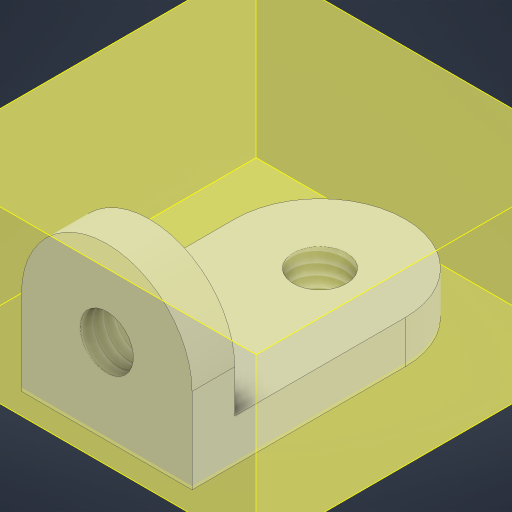
# Autodesk Inventor part: Rotational Linkage
Saved by Autodesk Inventor 2023 (Build 270158000, 158)
## iProperties
Created: 2022-05-02
Part Number: Rotational Linkage
Material: Generic
Document SubType Name: Modeling
Designer: FizzyApple12
Density: 1 g/cm^3
Appearance: Default
Author: FizzyApple12
Autodesk Inventor part; units mm, degrees
ref_plane "YZ Plane" through (0, 0, 0) normal (1, 0, 0) x (0, 1, 0)
ref_plane "XZ Plane" through (0, 0, 0) normal (0, 1, 0) x (-1, 0, 0)
ref_plane "XY Plane" through (0, 0, 0) normal (0, 0, 1) x (1, 0, 0)
sketch "Sketch1" plane through (0, 0, 0) normal (0, 1, 0) x (-1, 0, 0)
  circle A0 centre (0, 0) radius 6.35
  line L0 (6.35, 0) -> (6.35, 12.7)
  line L1 (6.35, 12.7) -> (-6.35, 12.7)
  line L2 (-6.35, 12.7) -> (-6.35, 0)
  dimension "d0" = 12.7
  dimension "d1" = 12.7
  constraints: 6 end point, 2 coincident, 2 point on circle, 2 tangent, 1 centre point, 1 parallel, 1 perpendicular, 1 vertical
  measures "d0" diameter of A0
  measures "d1" distance of L0.start L0.end
extrude "Extrusion1" add sketch "Sketch1" along normal blind 3.175
sketch "Sketch2" plane through (-6.35, 0, 12.7) normal (0, 0, 1) x (1, 0, 0)
  circle A0 centre (6.35, 6.35) radius 6.35
  line L0 (0, 6.35) -> (0, 0)
  line L1 (0, 0) -> (12.7, 0) projected
  line L2 (0, 0) -> (12.7, 0)
  line L3 (12.7, 0) -> (12.7, 6.35)
  point P0 (6.35, 0)
  dimension "d4" = 12.7
  dimension "d5" = 6.35
  constraints: 6 end point, 2 point on circle, 2 tangent, 1 centre point, 1 coincident, 1 perpendicular, 1 vertical
  measures "d4" diameter of A0
  measures "d5" distance from line of A0.centre L1
extrude "Extrusion2" add sketch "Sketch2" along normal blind 3.175
hole "Hole1" at (0, 0, 0) direction (0, 1, 0) diameter 3.9624 depth 13.6144 thread size "10-32 UNF" class "2B" standard "ANSI Unified Screw Threads"
hole "Hole2" at (0, 6.35, 12.7) direction (0, 0, 1) diameter 3.9624 end through all thread size "10-32 UNF" class "2B" standard "ANSI Unified Screw Threads"
body "Solid1"
